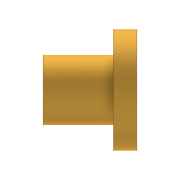
# Autodesk Inventor part: TR-20x4 nut
Saved by Autodesk Inventor 2020 (Build 240168000, 168)
## iProperties
Created: 2021-01-05
Part Number: TR-20x4 nut
Material: Brass, Soft Yellow
Document SubType Name: Modeling
Designer: John Knox R
Density: 8.47 g/cm^3
Appearance: Brass - Satin
Mass: 234.247 g
Surface Area: 113.345 cm^2
Volume: 27.6561 cm^3
Author: John Knox R
Autodesk Inventor part; units mm, degrees
ref_plane "YZ Plane" through (0, 0, 0) normal (1, 0, 0) x (0, 1, 0)
ref_plane "XZ Plane" through (0, 0, 0) normal (0, 1, 0) x (-1, 0, 0)
ref_plane "XY Plane" through (0, 0, 0) normal (0, 0, 1) x (1, 0, 0)
sketch "Sketch1" plane through (0, 0, 0) normal (0, 0, 1) x (1, 0, 0)
  circle A0 centre (0, 0) radius 26
  dimension "d4" = 52
  constraints: 1 centre point, 1 coincident
  measures "d4" diameter of A0
extrude "Extrusion1" add sketch "Sketch1" along normal blind 10
sketch "Sketch2" plane through (0, 0, 10) normal (0, 0, 1) x (1, 0, 0)
  circle A0 centre (0, 0) radius 15
  dimension "d5" = 30
  constraints: 1 centre point, 1 coincident
  measures "d5" diameter of A0
extrude "Extrusion2" add sketch "Sketch2" along normal blind 30
sketch "Sketch3" plane through (0, 0, 0) normal (0, 0, -1) x (-1, 0, 0)
  circle A0 centre (0, 0) radius 8.095
  dimension "d6" = 16.19
  constraints: 1 centre point, 1 coincident
  measures "d6" diameter of A0
extrude "Extrusion3" cut sketch "Sketch3" against normal through all
sketch "Sketch4" plane through (0, 0, 0) normal (0, 0, -1) x (-1, 0, 0)
  circle A0 centre (0, 0) radius 20 construction
  point P0 (20, 0)
  point P1 (0, 20)
  point P2 (-20, 0)
  point P3 (0, -20)
  dimension "d9" = 40
  dimension "d12" = 360
  constraints: 2 horizontal alignment, 1 coincident, 7 other
hole "Hole1" at (-20, 0, 0) at (0, 20, 0) at (20, 0, 0) at (0, -20, 0) direction (0, 0, 1) diameter 5.3 end through all clearance for "Socket Head Cap Screw" size "M5" standard "Ansi Metric M Profile"
sketch "Sketch5" plane through (0, 0, 0) normal (0, 0, -1) x (-1, 0, 0)
  circle A0 centre (20, 0) radius 2.65 construction
  point P0 (0, 0)
  constraints: 1 coincident
hole "Hole2" at (-20, 0, 0) direction (0, 0, 1) diameter 5.5 end through all counterbore diameter 10 counterbore depth 5.5 clearance for "Socket Head Cap Screw ISO 4762" size "M5" standard "ISO"
pattern_circular "Circular Pattern1" count 4 over 360 about axis through (0, 0, 0) along (0, 0, 1) of "Hole2"
sketch "Sketch12" plane through (0, 0, 0) normal (1, 0, 0) x (0, 1, 0)
  line L0 (0, -14.4529) -> (0, 43.8356)
  line L1 (8.095, 0) -> (8.095, 40) projected
  line L2 (8.095, 1.2666) -> (10.34, 0.6655)
  line L3 (10.34, 0.6655) -> (10.34, 0.0005)
  line L4 (10.34, 0.0005) -> (10.34, -0.6646)
  line L5 (10.34, -0.6646) -> (8.095, -1.2666)
  line L6 (8.095, 2) -> (8.095, 1.2666)
  line L7 (8.095, -1.2666) -> (8.095, -2)
  line L8 (8.095, 2) -> (8.095, -2)
  line L9 (8.095, -2) -> (0, -2)
  line L10 (0, -2) -> (0, 2)
  line L11 (0, 2) -> (8.095, 2)
  point P0 (0, 0)
  point P1 (0, 0)
  dimension "d69" = 4
  dimension "d70" = 8.095
  dimension "d71" = 8.095
  dimension "d72" = 4
  dimension "d73" = 0.6651
  dimension "d74" = 0.6651
  dimension "d75" = 0.602
  dimension "d76" = 0.7334
  dimension "d77" = 0.7334
  constraints: 22 end point, 1 midpoint, 1 vertical, 4 other
  measures "d69" distance of L9.end L10.end
  measures "d70" distance of L7.end L9.end
  measures "d71" distance of L10.end L6.start
  measures "d72" distance of L6.start L7.end
  measures "d73" distance of L3.end L2.end
  measures "d74" distance of L4.end L3.end
  measures "d75" vertical distance of L5.end L4.end
  measures "d76" distance of L6.start L2.start
  measures "d77" distance of L7.end L5.end
sketch "Sketch13" plane through (0, 0, 0) normal (0, 0, 1) x (1, 0, 0)
  point P0 (0, 0)
sketch "Sketch14" plane through (0, 0, 0) normal (1, 0, 0) x (0, 1, 0)
  line L0 (8.095, 2) -> (8.095, -2) projected
  line L1 (10.34, -0.6646) -> (8.095, -1.2666) projected
  line L2 (10.34, 0.0005) -> (10.34, -0.6646) projected
  line L3 (10.34, 0.6655) -> (10.34, 0.0005) projected
  line L4 (8.095, 1.2666) -> (10.34, 0.6655) projected
  line L5 (8.095, 2) -> (8.095, 1.2666) projected
  point P0 (0, 0)
coil "Coil2" sketch "Sketch14" operation cut axis through (0, 0, -14.4529) along (0, 0, 1) pitch 4 turns 12.5 hand left
coil "Coil3" sketch "Sketch14" operation cut axis through (0, 0, -10) along (0, 0, -1) pitch 4 turns 1.25 hand left
equation "\"D1\" = 22"
equation "\"D2\" = 32"
equation "\"D3\" = 45"
equation "\"Tr\" = 16"
body "Solid1"
